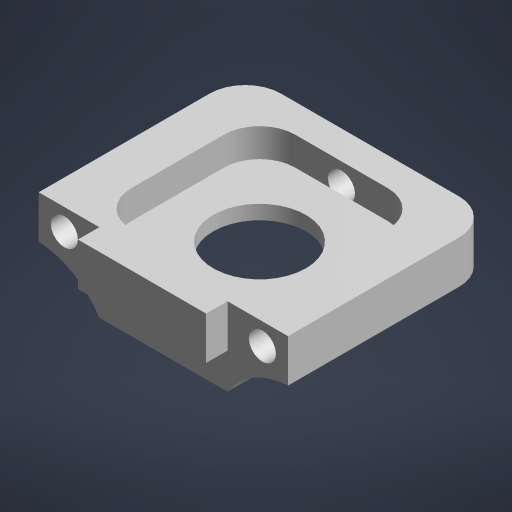
# Autodesk Inventor part: Endcap
Saved by Autodesk Inventor 2024.2 (Build 282272000, 272)
## iProperties
Part Number: Endcap
Material: ABS-Kunststoff
Document SubType Name: Modellieren
Designer: Timo de Vries
Appearance: Weiß
Mass: 28.9059 g
Surface Area: 30.6141 cm^2
Volume: 3.61324 cm^3
Density: 1.06 g/cm^3
Author: Timo de Vries
Autodesk Inventor part; units mm, degrees
ref_plane "YZ-Ebene" through (0, 0, 0) normal (1, 0, 0) x (0, 1, 0)
ref_plane "XZ-Ebene" through (0, 0, 0) normal (0, 1, 0) x (-1, 0, 0)
ref_plane "XY-Ebene" through (0, 0, 0) normal (0, 0, 1) x (1, 0, 0)
sketch "Skizze1" plane through (0, 0, 0) normal (0, 0, 1) x (1, 0, 0)
  line L0 (-17.5, 0) -> (-17.5, 29)
  line L1 (-17.5, 29) -> (17.5, 29)
  line L2 (17.5, 29) -> (17.5, 0)
  line L3 (17.5, 0) -> (9, 0)
  line L4 (9, 0) -> (9, -3)
  line L5 (9, -3) -> (-9, -3)
  line L6 (-9, -3) -> (-9, 0)
  line L7 (-9, 0) -> (-17.5, 0)
  point P0 (0, 0)
  point P1 (0, -3)
  point P2 (0, 29)
  point P3 (13.25, 0)
  dimension "d0" = 18
  dimension "d1" = 35
  dimension "d2" = 29
  dimension "d3" = 3
  constraints: 16 end point, 7 perpendicular, 3 midpoint, 2 vertical alignment, 1 horizontal alignment, 1 point on line, 1 vertical
  measures "d0" distance of L4.end L5.end
  measures "d1" distance of L0.end L1.end
  measures "d2" distance between parallel lines of L1 L3
  measures "d3" distance between parallel lines of L3 L5
extrude "Extrusion1" add sketch "Skizze1" along normal mid plane 6
sketch "Skizze2" plane through (0, 0, 3) normal (0, 0, 1) x (1, 0, 0)
  line L0 (-11.5, 25) -> (11.5, 25)
  line L1 (11.5, 25) -> (11.5, 2)
  line L2 (11.5, 2) -> (-11.5, 2)
  line L3 (-11.5, 2) -> (-11.5, 25)
  line L4 (-11.5, 25) -> (11.5, 2) construction
  line L5 (11.5, 25) -> (-11.5, 2) construction
  line L6 (-9, -3) -> (9, -3) projected
  point P0 (0, 0)
  point P1 (0, 13.5)
  point P2 (0, 2)
  dimension "d27" = 16.5
  dimension "d28" = 23
  constraints: 12 end point, 3 midpoint, 2 parallel, 2 perpendicular, 1 horizontal, 1 vertical alignment
  measures "d27" distance from line of L6 point (0, 13.5)
  measures "d28" distance of L0.start L0.end
extrude "Extrusion2" cut sketch "Skizze2" against normal blind 4
fillet "Rundung1" radius 5 6 edges at (-17.5, 29, 0) (17.5, 29, 0) (-11.5, 25, 1) (11.5, 25, 1) (11.5, 2, 1) (-11.5, 2, 1)
sketch "Skizze3" plane through (0, 0, -1) normal (0, 0, 1) x (1, 0, 0)
  circle A0 centre (0, 13.5) radius 6.5
  line L0 (-9, -3) -> (9, -3) construction
  line L1 (9, -3) -> (-9, -3) construction
  point P0 (0, 0)
  dimension "d12" = 13
  dimension "d13" = 16.5
  constraints: 1 centre point, 1 vertical alignment
  measures "d12" diameter of A0
  measures "d13" distance from line of A0.centre L0
extrude "Extrusion3" cut sketch "Skizze3" against normal through all
sketch "Skizze4" plane through (9, 0, 3) normal (0, -1, 0) x (1, 0, 0)
  line L0 (-22.9, -3) -> (-9, -3) construction
  line L1 (-9, -3) -> (4.9, -3) construction
  dimension "d19" = 27.8
  constraints: 4 end point, 2 collinear, 1 horizontal
  measures "d19" distance of L1.end L0.start
hole "Bohrung1" at (-13.9, 0, 0) at (13.9, 0, 0) direction (0, 1, 0) diameter 3.8 depth 8 tip angle 118
sketch "Skizze5" plane through (0, 0, -3) normal (0, 0, -1) x (-1, 0, 0)
  line L0 (-9, -3) -> (-9, 0) projected
  line L1 (-9, 0) -> (9, 0)
  line L2 (9, 0) -> (9, 5)
  line L3 (9, 5) -> (-9, 5)
  line L4 (-9, 5) -> (-9, 0)
  point P0 (0, 0)
  dimension "d29" = 5
  constraints: 8 end point, 2 parallel, 1 coincident, 1 horizontal, 1 perpendicular
  measures "d29" distance between parallel lines of L1 L3
extrude "Extrusion4" add sketch "Skizze5" along normal blind 5
fillet "Rundung2" radius 10.75 2 edges at (9, 2.5, -3) (-9, 2.5, -3)
sketch "Skizze6" plane through (-12.5, 29, -3) normal (0, 1, 0) x (1, 0, 0)
  point P0 (12.5, -3)
hole "Bohrung2" at (0, 29, 0) direction (0, -1, 0) diameter 3.8 depth 4
